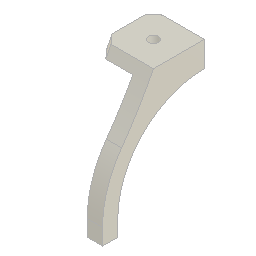
ptfe tube support v2 (Autodesk Fusion 360 design; units mm, degrees)
Autodesk Fusion 360 part; units mm, degrees
sketch "Sketch1" plane through (0, 0, 0) normal (0, 0, 1) x (1, 0, 0)
  line L0 (15, -15) -> (-15, -15)
  line L1 (-15, -15) -> (-15, 15)
  line L2 (-15, 15) -> (15, 15)
  line L3 (15, 15) -> (15, -15)
  line L4 (15, -15) -> (-15, 15) construction
  line L5 (-15, -15) -> (15, 15) construction
  circle A0 centre (0, 0) radius 3
  circle A1 centre (0, 0) radius 5.25 construction
  dimension "d1" = 30
  dimension "d2" = 30
  dimension "d3" = 6
  dimension "d22" = 10.5
  constraint horizontal L0
  constraint perpendicular L0 L1
  constraint parallel L0 L2
  constraint parallel L1 L3
  constraint coincident L4 A0.centre
  constraint coincident L5 A0.centre
  constraint coincident A0.centre A1.centre
  measures "d1" distance of L1.end L2.end
  measures "d2" distance of L0.end L1.end
  measures "d3" diameter of A0
  measures "d22" diameter of A1
extrude "Extrude1" add sketch "Sketch1" along normal blind 6 makes body 1
sketch "Sketch2" plane through (15, 0, 0) normal (1, 0, 0) x (0, 1, 0)
  line L0 (-15, 0) -> (15, 0)
  line L1 (15, 0) -> (15, 6)
  line L2 (15, 6) -> (-15, 6)
  line L3 (-15, 6) -> (-15, 0)
  arc A0 (15, 0) -> (-45, -60) centre (15, -60) ccw
  line L4 (-45, -60) -> (-45, -69.4872)
  dimension "d6" = 60
  constraint tangent L0 A0
  constraint coincident L0.end L1.start
  constraint vertical L4
  constraint tangent A0 L4
  measures "d6" radius of A0
sketch "Sketch3" plane through (0, 15, 0) normal (0, 1, 0) x (-1, 0, 0)
  line L0 (-15, 0) -> (15, 0)
  line L1 (15, 0) -> (15, 6)
  line L2 (15, 6) -> (-15, 6)
  line L3 (-15, 6) -> (-15, 0)
  circle A0 centre (-10.5, -4.5) radius 4.5
  line L4 (-6, -4.5) -> (-6, 0)
  line L5 (-15, -4.5) -> (-15, 0)
  line L6 (-10.5, -9) -> (-15, -9)
  line L7 (-15, -9) -> (-15, -4.5)
  line L8 (-7, -4.5) -> (-10.5, -8)
  line L9 (-10.5, -8) -> (-14, -4.5)
  line L10 (-14, -4.5) -> (-10.5, -1)
  line L11 (-10.5, -1) -> (-7, -4.5)
  line L12 (-10.5, -8) -> (-10.5, -1) construction
  point P0 (-15, 0)
  dimension "d17" = 9
  dimension "d18" = 7
  constraint coincident A0 L4.start
  constraint tangent A0 L4
  constraint coincident L0 L4.end
  constraint perpendicular L0 L4
  constraint coincident A0 L5.start
  constraint coincident L0 P0
  constraint perpendicular L0 L5
  constraint coincident P0 L0.start
  constraint tangent L0 A0
  constraint tangent A0 L5
  constraint coincident A0 L6.start
  constraint tangent A0 L6
  constraint horizontal L6
  constraint tangent A0 L7
  constraint perpendicular L8 L9
  constraint parallel L8 L10
  constraint parallel L9 L11
  constraint vertical L12
  constraint equal L8 L9
  constraint midpoint A0.centre L12
  measures "d17" diameter of A0
  measures "d18" distance of L8.end L10.end
sweep "Sweep1" add profiles "Sketch3" path "Sketch2" along A0 L4 section 1 contours L0 A0 L4 | L0 A0 L5 | A0 | A0 L6 L7 separate body makes body 2
sketch "Sketch4" plane through (0, 0, 0) normal (0, 0, -1) x (1, 0, 0)
  circle A0 centre (0, 0) radius 3
  line L0 (-15, -15) -> (15, -15)
  line L1 (15, -15) -> (15, 15)
  line L2 (15, 15) -> (-15, 15)
  line L3 (-15, 15) -> (-15, -15)
  line L4 (6, -15) -> (10.5, -15)
  arc A1 (6, 40.5) -> (10.5, 36) centre (10.5, 40.5) ccw
  line L5 (6, -15) -> (6, 40.5)
  line L6 (10.5, -15) -> (10.5, 36)
extrude "Extrude2" add sketch "Sketch4" along normal up to surface contours L0 L2 L4 L5 L6 | L0 L1 L2 L6 end surface at (9, -44.7283, -54.2966) on bodies 2 bodies 1 2
fillet "Fillet1" radius 229.426 1 edges at (10.5, -15, -8.0385) on bodies 1
chamfer "Chamfer1" distance 5 angle 45 2 edges at (-15, 15, 3) (-15, -16.5371, 2.9885) on bodies 1
